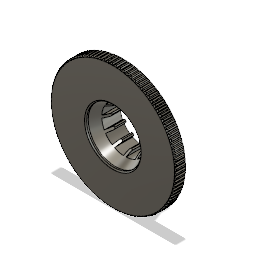
focus_ring (Autodesk Fusion 360 design; units mm, degrees)
Autodesk Fusion 360 part; units mm, degrees
sketch "Sketch1" plane through (0, 0, 0) normal (0, 0, 1) x (1, 0, 0)
  circle A0 centre (0, 0) radius 6.198
  circle A1 centre (0, 0) radius 7.4975
  dimension "d2" = 12.396
  dimension "d3" = 14.995
  measures "d2" diameter of A0
  measures "d3" diameter of A1
extrude "Extrude1" add sketch "Sketch1" along normal blind 2.7
sketch "Sketch2" plane through (0, 0, 2.7) normal (0, 0, 1) x (1, 0, 0)
  circle A0 centre (0, 0) radius 6.198
  circle A1 centre (0, 0) radius 7.4975
  circle A2 centre (0, 0) radius 7.5875
  circle A3 centre (0, 0) radius 6.198
  circle A4 centre (0, 0) radius 7.4975
  circle A5 centre (0, 0) radius 8.5875
  dimension "d6" = 15.175
  dimension "d19" = 1
  measures "d6" diameter of A2
extrude "Extrude2" add sketch "Sketch2" along normal blind 2.5 contours A1 A4 | A2
sketch "Sketch3" plane through (0, 0, 5.2) normal (0, 0, 1) x (1, 0, 0)
  circle A0 centre (0, 0) radius 6.198
  circle A1 centre (0, 0) radius 7.5875
  circle A2 centre (0, 0) radius 16.9975
  circle A3 centre (0, 0) radius 6.198
  dimension "d9" = 33.995
  measures "d9" diameter of A2
extrude "Extrude3" add sketch "Sketch3" along normal blind 3 contours A1 | A2
sketch "Sketch4" plane through (0, 0, 0) normal (0, 1, 0) x (1, 0, 0)
  line L0 (-16.9975, -5.2) -> (16.9975, -5.2)
  line L1 (8.5248, -5.2) -> (6.8311, -0.6214)
  line L2 (6.9882, -2.9263) -> (7.3, -5.2)
  line L3 (6.9882, -2.9263) -> (6.8311, -0.6214)
  dimension "d12" = 110.3
  measures "d12" angle of L0 L1
revolve "Revolve1" add sketch "Sketch4" angle 360 about axis through (0, 0, 1.75) along (0, 0, 1)
sketch "Sketch5" plane through (0, 0, 8.2) normal (0, 0, 1) x (1, 0, 0)
  circle A0 centre (0, 0) radius 6.198
  circle A1 centre (0, 0) radius 16.9975
  circle A2 centre (0, 0) radius 7.3635
  dimension "d14" = 14.727
  measures "d14" diameter of A2
extrude "Extrude4" cut sketch "Sketch5" against normal blind 0.7 contours A0 | A2
extrude "Extrude5" cut sketch "Sketch2" against normal blind 3.4 contours A2 | A5
sketch "Sketch7" plane through (0, 0, 0) normal (0, 0, -1) x (-1, 0, 0)
  circle A0 centre (0, 0) radius 6.198 construction
  circle A1 centre (0, 0) radius 7.4975
  line L0 (0, 2.5) -> (0, -8.8363) construction
  line L1 (-0.35, -5.298) -> (0.35, -5.298)
  line L2 (0.35, -5.298) -> (0.35, -7.0295)
  line L3 (0.35, -7.0295) -> (-0.35, -7.0295)
  line L4 (-0.35, -7.0295) -> (-0.35, -5.298)
  line L5 (-1.7511, -6.198) -> (2.0489, -6.198) construction
  circle A2 centre (0, 0) radius 7.4975 construction
  line L6 (-0.35, -5.473) -> (0.35, -5.473)
  spline S0 degree 5 poles (-0.35, -5.473) (-0.3457, -5.4599) (-0.3351, -5.4349) (-0.313, -5.4007) (-0.2713, -5.3619) (-0.1981, -5.3256) (-0.1061, -5.3026) (0, -5.2942) (0.1061, -5.3012) (0.1981, -5.3233) (0.2713, -5.3594) (0.313, -5.3988) (0.3351, -5.4338) (0.3457, -5.4595) (0.35, -5.473) knots 0 0 0 0 0 0 0.1 0.2 0.3 0.4 0.5 0.6 0.7 0.8 0.9 1 1 1 1 1 1
  line L7 (-0.0937, -5.2986) -> (0.0937, -5.2974)
  dimension "d22" = 0.7
  dimension "d23" = 0.35
  dimension "d24" = 0.9
  dimension "d27" = 0.175
  measures "d22" distance of L2 L4
  measures "d23" distance of L0 L4
  measures "d24" distance of L1 L5
  measures "d27" distance of L1 L6
extrude "Extrude6" add sketch "Sketch7" against normal blind 7.5 contours L2 L3 L4 L6 | L1 L6 S0 L7
pattern_circular "C-Pattern1" count 12 over 360 about axis through (0, 0, 1.75) along (0, 0, 1) of "Extrude6"
sketch "Sketch6" plane through (0, 0, 0) normal (0, 1, 0) x (1, 0, 0)
  line L0 (-5.8184, -4.1865) -> (-7.3635, -7.5)
  line L1 (-16.9975, -8.2) -> (16.9975, -8.2)
  line L2 (-7.3635, -7.5) -> (-7.3635, -7.9)
  line L3 (-7.3635, -7.9) -> (-7.6353, -7.8558)
  line L4 (-7.6353, -7.8558) -> (-7.5518, -6.9177)
  line L5 (-7.5518, -6.9177) -> (-6.198, -4.7846)
  line L6 (-6.198, -4.7846) -> (-6.1982, -5.0011)
  line L7 (-7.3635, -7.5) -> (-7.3635, -7.9)
  line L8 (-5.6408, -7.9) -> (-7.3635, -7.9)
  line L9 (-5.8184, -4.1865) -> (-4.4844, -1.3258)
  line L10 (-4.4844, -1.3258) -> (-3.6, -7.9)
  line L11 (-3.6, -7.9) -> (-5.6408, -7.9)
  dimension "d20" = 155
  measures "d20" angle of L0 L2
revolve "Revolve2" cut sketch "Sketch6" angle 360 about axis through (0, 0, 1.75) along (0, 0, 1) contours L0 L2 L7 L8 L9 L10 L11
chamfer "Chamfer1" distance 0.3 angle 45 1 edges at (-6.9901, -2.7112, 0)
chamfer "Chamfer2" distance 0.3 angle 45 1 edges at (-6.8652, 2.6628, 8.2)
sketch "Sketch8" plane through (0, 0, 8.2) normal (0, 0, 1) x (1, 0, 0)
  circle A0 centre (0, 0) radius 16.9975
  circle A1 centre (0, 0) radius 7.6635
  line L0 (-0.5, 17.25) -> (0.5, 17.25)
  line L1 (0.5, 17.25) -> (0.1536, 16.65)
  line L2 (-0.1536, 16.65) -> (-0.5, 17.25)
  line L3 (-0.1536, 16.65) -> (0.1536, 16.65)
  line L4 (0, 16.384) -> (-0.1536, 16.65) construction
  line L5 (0.1536, 16.65) -> (0, 16.384) construction
  dimension "d32" = 1
  dimension "d36" = 1
  dimension "d37" = 1
  dimension "d38" = 60
  measures "d38" angle of L1 L2
chamfer "Chamfer3" distance 0.3 angle 45 2 edges at (-15.8472, -6.1466, 8.2) (-15.8472, -6.1466, 5.2)
extrude "Extrude7" cut sketch "Sketch8" against normal blind 3 contours A0 L1 L2 L3 | A0 L0 L1 L2 picked at (0.0391, 16.7657)
pattern_circular "C-Pattern2" count 100 over 360 about axis through (0, 0, 1.75) along (0, 0, 1) of "Extrude7"
equation "d23 = 0.70 mm / 2"
named bodies: "Focus Ring"
